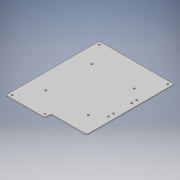
# Autodesk Inventor part: bottomMountingPlate2
Saved by Autodesk Inventor 2018 (Build 220112000, 112)
## iProperties
Created: 2020-02-26
Part Number: bottomMountingPlate2
Material: Generic
Document SubType Name: Modeling
Designer: anirudh
Density: 1 g/cm^3
Appearance: Default
Author: anirudh
Autodesk Inventor part; units mm, degrees
ref_plane "YZ Plane" through (0, 0, 0) normal (1, 0, 0) x (0, 1, 0)
ref_plane "XZ Plane" through (0, 0, 0) normal (0, 1, 0) x (-1, 0, 0)
ref_plane "XY Plane" through (0, 0, 0) normal (0, 0, 1) x (1, 0, 0)
sketch "Sketch1" plane through (0, 0, 0) normal (0, 1, 0) x (-1, 0, 0)
  line L0 (50.4698, -94.8182) -> (63.1698, -94.8182)
  line L1 (63.1698, -94.8182) -> (63.1698, -82.1182)
  line L2 (50.4698, 94.8182) -> (63.1698, 94.8182)
  line L3 (63.1698, 94.8182) -> (63.1698, 82.1182)
  circle A0 centre (56.8198, 88.4682) radius 1.75
  circle A1 centre (56.8198, -88.4682) radius 1.75
  circle A2 centre (-82.2198, -88.4682) radius 1.75
  line L4 (-15.875, 82.1182) -> (-15.875, 94.8182)
  line L5 (-15.875, 94.8182) -> (-3.175, 94.8182)
  circle A3 centre (-9.525, 88.4682) radius 1.75
  line L6 (-15.875, 94.8182) -> (63.1698, 94.8182)
  line L7 (63.1698, 94.8182) -> (63.1698, -94.8182)
  line L8 (63.1698, -94.8182) -> (-88.5698, -94.8182)
  line L9 (-15.875, 82.1182) -> (-88.5698, 82.1182)
  line L10 (-88.5698, -94.8182) -> (-88.5698, 82.1182)
  circle A4 centre (-56.047, -46.609) radius 1.75
  circle A5 centre (-56.047, -46.609) radius 1.75
  circle A6 centre (30.647, -46.609) radius 1.75
  circle A7 centre (30.647, -46.609) radius 1.75
  circle A8 centre (30.647, 46.609) radius 1.75
  circle A9 centre (30.647, 46.609) radius 1.75
  circle A10 centre (-56.047, 46.609) radius 1.75
  circle A11 centre (-56.047, 46.609) radius 1.75
  point P0 (15.9004, 85.2932)
  point P1 (63.1698, 85.2932)
  point P2 (63.1698, -85.2932)
  constraints: 22 end point, 12 centre point, 4 coincident, 1 horizontal, 1 perpendicular
extrude "Extrusion1" add sketch "Sketch1" along normal blind 1.5875
fillet "Fillet1" radius 3.175 6 edges at (-63.1698, 0.7937, 94.8182) (15.875, 0.7937, 94.8182) (15.875, 0.7937, 82.1182) (88.5698, 0.7937, 82.1182) (88.5698, 0.7937, -94.8182) (-63.1698, 0.7937, -94.8182)
sketch "Sketch2" plane through (0, 1.5875, 0) normal (0, 1, 0) x (1, 0, 0)
  line L0 (-63.1698, 91.6432) -> (-63.1698, -91.6432) projected
  arc A0 (-59.9948, 94.8182) -> (-63.1698, 91.6432) centre (-59.9948, 91.6432) ccw projected
  line L1 (-63.1698, 91.6432) -> (-63.1698, -91.6432)
  line L2 (88.5698, -78.9432) -> (88.5698, 91.6432) projected
  line L3 (69.5198, 0) -> (69.5198, -38.1)
  line L4 (69.5198, -38.1) -> (88.5698, -38.1)
  line L5 (88.5698, -38.1) -> (88.5698, 0)
  line L6 (88.5698, -38.1) -> (69.5198, -38.1)
  line L7 (69.5198, -38.1) -> (69.5198, 38.1)
  line L8 (69.5198, 38.1) -> (88.5698, 38.1)
  line L9 (88.5698, 38.1) -> (88.5698, -38.1)
  line L10 (69.5198, -38.1) -> (88.5698, -38.1)
  line L11 (88.5698, -38.1) -> (88.5698, -19.05)
  line L12 (69.5198, -19.05) -> (69.5198, -38.1)
  circle A1 centre (79.0448, -28.575) radius 1.75
  line L13 (69.5198, 38.1) -> (88.5698, 38.1)
  line L14 (88.5698, 38.1) -> (88.5698, 19.05)
  line L15 (69.5198, 19.05) -> (69.5198, 38.1)
  circle A2 centre (79.0448, 28.575) radius 1.75
  circle A3 centre (79.0448, -18.415) radius 1.75
  circle A4 centre (79.0448, 18.415) radius 1.75
  point P0 (0, 0)
  dimension "d3" = 19.05
  dimension "d7" = 19.05
  dimension "d8" = 3.5
  dimension "d9" = 19.05
  dimension "d10" = 3.5
  dimension "d15" = 3.5
  dimension "d16" = 3.5
  constraints: 28 end point, 6 equal length, 4 centre point, 3 horizontal, 3 perpendicular, 3 point on line
  measures "d3" distance of L4.end L3.end
  measures "d7" distance of L11.end L10.end
  measures "d8" diameter of A1
  measures "d9" distance of L13.end L14.end
  measures "d10" diameter of A2
  measures "d15" diameter of A3
  measures "d16" diameter of A4
extrude "Extrusion3" cut sketch "Sketch2" against normal blind 25.4 contours A1 | A2 | A3 | A4
body "Solid1"
